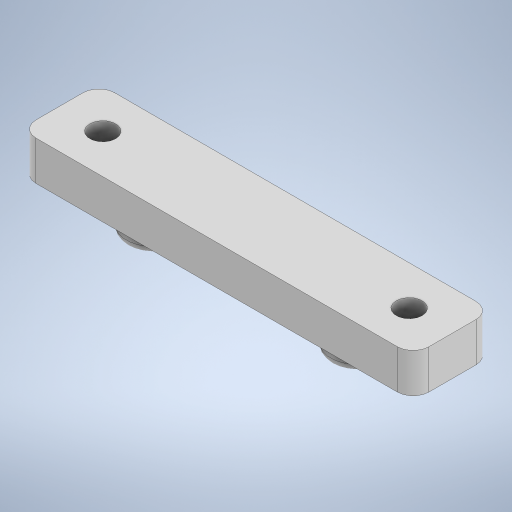
# Autodesk Inventor part: Shablon2
Saved by Autodesk Inventor 2024 (Build 280153000, 153)
## iProperties
Created: 2023-11-28
Part Number: Shablon2
Material: Типовые
Document SubType Name: Modeling
Designer: fm
Density: 1 g/cm^3
Appearance: По умолчанию
Author: fm
Autodesk Inventor part; units mm, degrees
ref_plane "YZ Plane" through (0, 0, 0) normal (1, 0, 0) x (0, 1, 0)
ref_plane "XZ Plane" through (0, 0, 0) normal (0, 1, 0) x (-1, 0, 0)
ref_plane "XY Plane" through (0, 0, 0) normal (0, 0, 1) x (1, 0, 0)
sketch "Эскиз1" plane through (0, 0, 0) normal (0, 1, 0) x (-1, 0, 0)
  circle A0 centre (0, 0) radius 3.5
  circle A1 centre (-26, 0) radius 3.5
  line L0 (-3.5, 0) -> (-22.5, 0) construction
  line L1 (0, 0) -> (-26, 0) construction
  circle A2 centre (-32.5, 0) radius 1.65
  circle A3 centre (6.5, 0) radius 1.65
  line L2 (10, -5) -> (-36, -5)
  line L3 (-38, -3) -> (-38, 3)
  line L4 (-36, 5) -> (10, 5)
  line L5 (12, 3) -> (12, -3)
  arc A4 (10, -5) -> (12, -3) centre (10, -3) ccw
  arc A5 (12, 3) -> (10, 5) centre (10, 3) ccw
  arc A6 (-38, -3) -> (-36, -5) centre (-36, -3) ccw
  arc A7 (-36, 5) -> (-38, 3) centre (-36, 3) ccw
  circle A8 centre (-32.5, 0) radius 3.65
  circle A9 centre (6.5, 0) radius 3.65
  point P0 (3.5, 0)
  point P1 (4.85, 0)
  point P2 (-29.5, 0)
  point P3 (-30.85, 0)
  point P4 (-29.5, 0)
  point P5 (-30.85, 0)
  point P6 (-29.5, 0)
  point P7 (-30.85, 0)
  point P8 (-29.5, 0)
  point P9 (-30.85, 0)
  dimension "d4" = 3.3
  dimension "d5" = 3.3
  dimension "d0" = 7
  dimension "d1" = 7
  dimension "d3" = 19
  dimension "d8" = 3
  dimension "d9" = 3
  dimension "d10" = 12
  dimension "d11" = 12
  dimension "d12" = 5
  dimension "d13" = 10
  dimension "d14" = 2
  dimension "d15" = 2
  dimension "d16" = 2
  constraints: 13 point on circle, 12 end point, 8 centre point, 8 tangent, 6 coincident, 3 equal radius, 3 horizontal, 2 horizontal alignment, 2 parallel, 1 perpendicular, 1 point on line, 4 other
  measures "d0" diameter of A0
  measures "d1" diameter of A1
  measures "d3" distance of L0.start L0.end
  measures "d8" distance of point (-29.5, 0) A8.centre
  measures "d9" distance of A0.end A9.centre
  measures "d10" distance from line of L5 point (0, 0)
  measures "d11" distance from line of L3 L1.end
  measures "d12" distance from line of L2 L1.end
  measures "d13" distance between parallel lines of L2 L4
  measures "d14" radius of A4
extrude "Выдавливание1" add sketch "Эскиз1" along normal blind 5 contours A0 A9 | A0 A9 | A9 A0 | A1 A8 | A8 A1 | A1 A8 | L2 A6 L3 A7 L4 A5 L5 A4
extrude "Выдавливание2" add sketch "Эскиз1" against normal blind 3 contours A0 A9 | A9 A0 | A1 A8 | A8 A1 picked at (3.0809, 0.424) picked at (-1.3483, -0.2837) picked at (-24.6517, 0.2837) picked at (-29.2672, -0.4241)
fillet "Сопряжение1" radius 1 2 edges at (3.5, -3, 0) (29.5, -3, 0)
